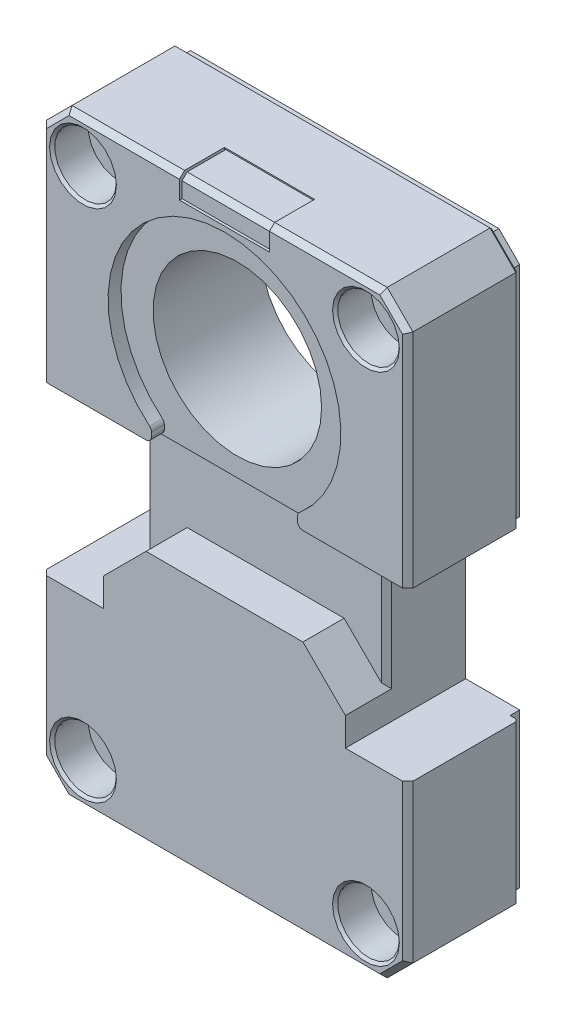
# Autodesk Inventor part: XM430_HOUSING_BOTTOM
Saved by Autodesk Inventor 2019.4 (Build 234330000, 330)
## iProperties
Created: 2019-12-10
Part Number: XM430_HOUSING_BOTTOM
Material: 一般
Document SubType Name: Modeling
Designer: y6tada
Density: 1 g/cm^3
Appearance: 既定
Author: y6tada
Autodesk Inventor part; units mm, degrees
ref_plane "YZ Plane" through (0, 0, 0) normal (1, 0, 0) x (0, 1, 0)
ref_plane "XZ Plane" through (0, 0, 0) normal (0, 1, 0) x (-1, 0, 0)
ref_plane "XY Plane" through (0, 0, 0) normal (0, 0, 1) x (1, 0, 0)
sketch "スケッチ1" plane through (0, 0, 0) normal (0, 0, 1) x (1, 0, 0)
  line L0 (-12.25, 11.25) -> (12.25, 11.25)
  line L1 (14.25, 9.25) -> (14.25, -33.25)
  line L2 (12.25, -35.25) -> (-12.25, -35.25)
  line L3 (-14.25, -33.25) -> (-14.25, 9.25)
  line L4 (-12.25, 11.25) -> (-14.25, 9.25)
  line L5 (12.25, 11.25) -> (14.25, 9.25)
  line L6 (14.25, -33.25) -> (12.25, -35.25)
  line L7 (-12.25, -35.25) -> (-14.25, -33.25)
  line L8 (0, 0) -> (0, -44.2059) construction
  line L9 (-11, 8) -> (11, 8) construction
  line L10 (11, 8) -> (11, -32) construction
  line L11 (11, -32) -> (-11, -32) construction
  line L12 (-11, -32) -> (-11, 8) construction
  circle A0 centre (0, 0) radius 6.55
  point P0 (-14.25, 11.25)
  point P1 (14.25, -35.25)
  point P2 (14.25, 11.25)
  point P3 (-14.25, -35.25)
  dimension "d0" = 2
  dimension "d1" = 2
  dimension "d2" = 2
  dimension "d3" = 2
  dimension "d4" = 2
  dimension "d5" = 2
  dimension "d6" = 2
  dimension "d7" = 2
  dimension "d8" = 28.5
  dimension "d9" = 46.5
  dimension "d10" = 11.25
  dimension "d11" = 8
  dimension "d12" = 22
  dimension "d13" = 40
  dimension "d29" = 13.1
  constraints: 26 end point, 8 point on line, 5 coincident, 4 parallel, 2 horizontal, 2 perpendicular, 1 centre point, 1 vertical, 2 other
  measures "d0" distance of L0.start point (-14.25, 11.25)
  measures "d1" distance of L3.end point (-14.25, 11.25)
  measures "d2" distance of L0.end point (14.25, 11.25)
  measures "d3" distance of L1.start point (14.25, 11.25)
  measures "d4" distance of L1.end point (14.25, -35.25)
  measures "d5" distance of L2.start point (14.25, -35.25)
  measures "d6" distance of L2.end point (-14.25, -35.25)
  measures "d7" distance of L3.start point (-14.25, -35.25)
  measures "d8" distance between parallel lines of L1 L3
  measures "d9" distance between parallel lines of L0 L2
  measures "d10" distance from line of L0 L8.start
  measures "d11" distance from line of L9 L8.start
  measures "d12" distance between parallel lines of L10 L12
  measures "d13" distance of L9.end L10.end
  measures "d29" diameter of A0
extrude "押し出し1" add sketch "スケッチ1" along normal blind 9.35
sketch "スケッチ2" plane through (0, 0, 9.35) normal (0, 0, 1) x (1, 0, 0)
  line L0 (11, 8) -> (-11, 8) construction
  line L1 (-11, 8) -> (-11, -32) construction
  line L2 (-11, -32) -> (11, -32) construction
  line L3 (11, -32) -> (11, 8) construction
  line L4 (0, 0) -> (0, -37.3392) construction
  dimension "d16" = 22
  dimension "d17" = 8
  dimension "d18" = 40
  constraints: 10 end point, 4 coincident, 2 parallel, 1 horizontal, 1 perpendicular, 1 vertical, 1 other
  measures "d16" distance of L1.end L2.end
  measures "d17" distance from line of L4.start L0
  measures "d18" distance of L2.end L0.start
hole "穴1" at (11, 8, 9.35) at (-11, 8, 9.35) at (-11, -32, 9.35) at (11, -32, 9.35) direction (0, 0, -1) diameter 2.5 end through all counterbore diameter 4.8 counterbore depth 2.8 clearance for "Socket Head Cap Screw ISO 4762" size "M2.5" standard "ISO"
sketch "スケッチ3" plane through (0, 0, 0) normal (0, 0, -1) x (-1, 0, 0)
  line L0 (12.25, 11.25) -> (14.25, 9.25) projected
  line L1 (-12.25, 11.25) -> (12.25, 11.25) projected
  line L2 (-14.25, 9.25) -> (-12.25, 11.25) projected
  line L3 (-14.25, -33.25) -> (-14.25, 9.25) projected
  line L4 (-12.25, -35.25) -> (-14.25, -33.25) projected
  line L5 (12.25, -35.25) -> (-12.25, -35.25) projected
  line L6 (14.25, -33.25) -> (12.25, -35.25) projected
  line L7 (14.25, 9.25) -> (14.25, -33.25) projected
  line L8 (13.6, -32.9808) -> (11.9808, -34.6)
  line L9 (11.9808, -34.6) -> (-11.9808, -34.6)
  line L10 (-11.9808, -34.6) -> (-13.6, -32.9808)
  line L11 (-13.6, -32.9808) -> (-13.6, 8.9808)
  line L12 (-13.6, 8.9808) -> (-11.9808, 10.6)
  line L13 (-11.9808, 10.6) -> (11.9808, 10.6)
  line L14 (11.9808, 10.6) -> (13.6, 8.9808)
  line L15 (13.6, 8.9808) -> (13.6, -32.9808)
  point P0 (0, 0)
  dimension "d26" = 0.65
  constraints: 16 end point, 7 other
  measures "d26" distance between parallel lines of L7 L15
extrude "押し出し2" cut sketch "スケッチ3" against normal blind 0.75
sketch "スケッチ4" plane through (0, 0, 9.35) normal (0, 0, 1) x (1, 0, 0)
  line L0 (-14.25, 9.25) -> (-14.25, -33.25) construction
  line L1 (14.25, -21) -> (9.4, -21)
  line L2 (-14.25, -21) -> (-14.25, -8)
  line L3 (-14.25, -8) -> (14.25, -8)
  line L4 (14.25, -8) -> (14.25, -21)
  line L5 (9.4, -21) -> (9.4, -18.8)
  line L6 (6.1, -15.5) -> (-6.1, -15.5)
  line L7 (-9.4, -18.8) -> (-9.4, -21)
  line L8 (0, 0) -> (0, -25.5974) construction
  line L9 (14.25, -33.25) -> (14.25, 9.25) construction
  line L10 (9.4, -18.8) -> (6.1, -15.5)
  line L11 (-6.1, -15.5) -> (-9.4, -18.8)
  line L12 (-9.4, -21) -> (-14.25, -21)
  line L13 (9.4, -21) -> (-9.4, -21) construction
  line L14 (12.25, 11.25) -> (-12.25, 11.25) construction
  point P0 (9.4, -15.5)
  point P1 (-9.4, -15.5)
  dimension "d30" = 3.3
  dimension "d31" = 3.3
  dimension "d32" = 3.3
  dimension "d33" = 3.3
  dimension "d34" = 4.85
  dimension "d35" = 19.25
  dimension "d36" = 32.25
  dimension "d37" = 5.5
  constraints: 24 end point, 5 parallel, 5 point on line, 4 horizontal, 3 perpendicular, 2 vertical, 1 collinear, 1 other
  measures "d30" distance of L5.end point (9.4, -15.5)
  measures "d31" distance of L6.start point (9.4, -15.5)
  measures "d32" distance of L6.end point (-9.4, -15.5)
  measures "d33" distance of L7.start point (-9.4, -15.5)
  measures "d34" distance between parallel lines of L0 L7
  measures "d35" distance between parallel lines of L3 L14
  measures "d36" distance between parallel lines of L14 L1
  measures "d37" distance between parallel lines of L1 L6
extrude "押し出し3" cut sketch "スケッチ4" against normal blind 3.2
sketch "スケッチ5" plane through (0, 0, 6.15) normal (0, 0, 1) x (1, 0, 0)
  line L0 (9.4, -21) -> (9.4, -18.8) projected
  line L1 (14.25, -8) -> (14.25, -21) projected
  line L2 (9.4, -21) -> (14.25, -21)
  line L3 (14.25, -21) -> (14.25, -8)
  line L4 (14.25, -8) -> (9.4, -8)
  line L5 (9.4, -8) -> (9.4, -21)
  line L6 (-9.4, -18.8) -> (-9.4, -21) projected
  line L7 (-14.25, -21) -> (-14.25, -8) projected
  line L8 (-9.4, -21) -> (-14.25, -21)
  line L9 (-14.25, -21) -> (-14.25, -8)
  line L10 (-14.25, -8) -> (-9.4, -8)
  line L11 (-9.4, -8) -> (-9.4, -21)
  point P0 (0, 0)
  constraints: 16 end point, 4 parallel, 2 horizontal, 2 perpendicular
extrude "押し出し4" cut sketch "スケッチ5" against normal through all
sketch "スケッチ6" plane through (0, 0, 9.35) normal (0, 0, 1) x (1, 0, 0)
  arc A0 (5.675, -7.0496) -> (-5.675, -7.0496) centre (0, 0) ccw
  line L0 (-9.4, -8) -> (9.4, -8) construction
  line L1 (-5.675, -7.0496) -> (5.675, -7.0496) construction
  line L2 (5.675, -7.0496) -> (5.675, -8)
  line L3 (5.675, -8) -> (-5.675, -8)
  line L4 (-5.675, -8) -> (-5.675, -7.0496)
  arc A1 (-5.675, -7.0496) -> (5.675, -7.0496) centre (0, 0) ccw construction
  dimension "d42" = 9.05
  dimension "d43" = 11.35
  constraints: 8 end point, 4 point on circle, 2 centre point, 2 parallel, 1 coincident, 1 horizontal, 1 perpendicular, 1 point on line
  measures "d42" radius of A0
  measures "d43" distance between parallel lines of L2 L4
extrude "押し出し5" cut sketch "スケッチ6" against normal blind 1
sketch "スケッチ7" plane through (0, 0, 9.35) normal (0, 0, 1) x (1, 0, 0)
  line L0 (12.25, 11.25) -> (-12.25, 11.25) construction
  line L1 (3.5, 11.25) -> (-3.5, 11.25)
  line L2 (-3.5, 11.25) -> (-3.5, 9.45)
  line L3 (-3.5, 9.45) -> (3.5, 9.45)
  line L4 (3.5, 9.45) -> (3.5, 11.25)
  line L5 (0, 0) -> (0, 9.45) construction
  dimension "d46" = 1.8
  dimension "d47" = 7
  constraints: 10 end point, 2 parallel, 1 horizontal, 1 midpoint, 1 perpendicular, 1 point on line, 1 vertical
  measures "d46" distance between parallel lines of L3 L0
  measures "d47" distance between parallel lines of L2 L4
extrude "押し出し6" cut sketch "スケッチ7" against normal blind 3.5
fillet "フィレット1" radius 0.4 4 edges at (-5.675, -8, 8.85) (-5.675, -7.0496, 8.85) (5.675, -7.0496, 8.85) (5.675, -8, 8.85)
chamfer "面取り1" distance 0.4 angle 45 13 edges at (-14.25, 0.625, 9.35) (-13.25, 10.25, 9.35) (-7.875, 11.25, 9.35) (7.875, 11.25, 9.35) (13.25, 10.25, 9.35) (14.25, 0.625, 9.35) (14.25, -27.125, 9.35) (13.25, -34.25, 9.35) (0, -35.25, 9.35) (-13.25, -34.25, 9.35) (-14.25, -27.125, 9.35) (-9.4, -13.4, 6.15) (9.4, -13.4, 6.15)
chamfer "面取り2" distance 0.2 angle 45 14 edges at (-14.25, 0.625, 0.75) (-13.25, 10.25, 0.75) (0, 11.25, 0.75) (13.25, 10.25, 0.75) (14.25, 0.625, 0.75) (14.25, -27.125, 0.75) (13.25, -34.25, 0.75) (0, -35.25, 0.75) (-13.25, -34.25, 0.75) (-14.25, -27.125, 0.75) (-11, 10.4, 9.35) (11, 10.4, 9.35) (11, -29.6, 9.35) (-11, -29.6, 9.35)
sketch "スケッチ8" plane through (0, 0, 5.85) normal (0, 0, 1) x (1, 0, 0)
  line L0 (3.4, 11.15) -> (-3.4, 11.15)
  line L1 (-3.4, 11.15) -> (-3.4, 9.55)
  line L2 (-3.4, 9.55) -> (3.4, 9.55)
  line L3 (3.4, 9.55) -> (3.4, 11.15)
  line L4 (-3.5, 11.25) -> (3.5, 11.25) construction
  line L5 (0, 0) -> (0, 9.55) construction
  dimension "d57" = 0.1
  dimension "d58" = 6.8
  dimension "d59" = 1.6
  constraints: 10 end point, 2 parallel, 1 horizontal, 1 midpoint, 1 perpendicular, 1 vertical
  measures "d57" distance between parallel lines of L0 L4
  measures "d58" distance of L0.start L0.end
  measures "d59" distance between parallel lines of L2 L0
extrude "押し出し7" add sketch "スケッチ8" along normal blind 3.4
chamfer "面取り3" distance 0.4 angle 45 1 edges at (0, 11.15, 9.25)
equation "\"d1\" = d0"
equation "\"d2\" = d0"
equation "\"d3\" = d2"
equation "\"d4\" = d0"
equation "\"d5\" = d4"
equation "\"d6\" = d0"
equation "\"d7\" = d6"
equation "\"d31\" = d30"
equation "\"d32\" = d30"
equation "\"d33\" = d32"
